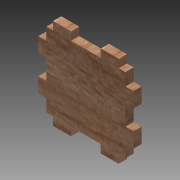
# Autodesk Inventor part: holder_plate_side
Saved by Autodesk Inventor 2015 (Build 190159000, 159)
## iProperties
Created: 2013-12-29
Part Number: holder_plate_side
Material: Wood (Birch)
Document SubType Name: Modeling
Designer: aoki
Density: 1 g/cm^3
Appearance: Birch - Natural Polished
Author: aoki
Autodesk Inventor part; units mm, degrees
ref_plane "YZ Plane" through (0, 0, 0) normal (1, 0, 0) x (0, 1, 0)
ref_plane "XZ Plane" through (0, 0, 0) normal (0, 1, 0) x (-1, 0, 0)
ref_plane "XY Plane" through (0, 0, 0) normal (0, 0, 1) x (1, 0, 0)
sketch "Block1" plane through (0, 0, 0) normal (0, 0, 1) x (1, 0, 0)
  line L0 (-35.5, -12.8333) -> (-26.5, -12.8333)
  line L1 (-30, 3.8333) -> (-35.5, 3.8333)
  line L2 (-35.5, 3.8333) -> (-26.5, 3.8333)
  line L3 (-26.5, 3.8333) -> (-26.5, -12.8333)
  line L4 (-26.5, -12.8333) -> (-35.5, -12.8333)
  line L5 (-35.5, -12.8333) -> (-35.5, 3.8333)
  line L6 (26.5, 3.8333) -> (35.5, 3.8333)
  line L7 (35.5, 3.8333) -> (26.5, 3.8333)
  line L8 (26.5, 3.8333) -> (26.5, -12.8333)
  line L9 (35.5, -12.8333) -> (35.5, 3.8333)
  line L10 (26.5, -12.8333) -> (35.5, -12.8333)
  line L11 (35.5, -12.8333) -> (26.5, -12.8333)
  point P0 (0, -4.5)
  dimension "d37" = 5.5
  measures "d37" distance of L1.start L1.end
sketch "Block2" plane through (0, 0, 0) normal (0, 0, 1) x (1, 0, 0)
  line L0 (-30, -5) -> (-35.5, -5)
  line L1 (-26.5, 5) -> (-35.5, 5)
  line L2 (-35.5, -5) -> (-26.5, -5)
  line L3 (-26.5, -5) -> (-26.5, 5)
  line L4 (-26.5, 5) -> (-35.5, 5)
  line L5 (-35.5, 5) -> (-35.5, -5)
  line L6 (26.5, -5) -> (26.5, 5)
  line L7 (35.5, -5) -> (26.5, -5)
  line L8 (26.5, 5) -> (35.5, 5)
  line L9 (35.5, 5) -> (35.5, -5)
  line L10 (26.5, 5) -> (35.5, 5)
  line L11 (26.5, -5) -> (35.5, -5)
  point P0 (0, 0)
  dimension "d51" = 5.5
  measures "d51" distance of L0.start L0.end
sketch "Block3" plane through (0, 0, 0) normal (0, 0, 1) x (1, 0, 0)
  line L0 (-9.9, 25.1) -> (9.9, 25.1)
  line L1 (9.9, 25.1) -> (9.9, 34.1)
  line L2 (9.9, 34.1) -> (22.1, 34.1)
  line L3 (22.1, 34.1) -> (22.1, 25.1)
  line L4 (22.1, 25.1) -> (26.6, 25.1)
  line L5 (26.6, 25.1) -> (26.6, 16.7667)
  line L6 (26.6, 16.7667) -> (35.6, 16.7667)
  line L7 (35.6, 16.7667) -> (35.6, 6.5667)
  line L8 (35.6, 6.5667) -> (26.6, 6.5667)
  line L9 (26.6, 6.5667) -> (26.6, -6.5667)
  line L10 (26.6, -6.5667) -> (35.6, -6.5667)
  line L11 (35.6, -6.5667) -> (35.6, -16.7667)
  line L12 (35.6, -16.7667) -> (26.6, -16.7667)
  line L13 (26.6, -16.7667) -> (26.6, -25.1)
  line L14 (26.6, -25.1) -> (22.1, -25.1)
  line L15 (22.1, -25.1) -> (22.1, -34.1)
  line L16 (22.1, -34.1) -> (9.9, -34.1)
  line L17 (9.9, -34.1) -> (9.9, -25.1)
  line L18 (9.9, -25.1) -> (-9.9, -25.1)
  line L19 (-9.9, -25.1) -> (-9.9, -34.1)
  line L20 (-9.9, -34.1) -> (-22.1, -34.1)
  line L21 (-22.1, -34.1) -> (-22.1, -25.1)
  line L22 (-22.1, -25.1) -> (-26.6, -25.1)
  line L23 (-26.6, -25.1) -> (-26.6, -16.7667)
  line L24 (-26.6, -16.7667) -> (-35.6, -16.7667)
  line L25 (-35.6, -16.7667) -> (-35.6, -6.5667)
  line L26 (-35.6, -6.5667) -> (-26.6, -6.5667)
  line L27 (-26.6, -6.5667) -> (-26.6, 6.5667)
  line L28 (-26.6, 6.5667) -> (-35.6, 6.5667)
  line L29 (-35.6, 6.5667) -> (-35.6, 16.7667)
  line L30 (-35.6, 16.7667) -> (-26.6, 16.7667)
  line L31 (-26.6, 16.7667) -> (-26.6, 25.1)
  line L32 (-26.6, 25.1) -> (-22.1, 25.1)
  line L33 (-22.1, 25.1) -> (-22.1, 34.1)
  line L34 (-22.1, 34.1) -> (-9.9, 34.1)
  line L35 (-9.9, 34.1) -> (-9.9, 25.1)
  line L36 (-26.5, -6.6667) -> (-35.5, -6.6667)
  line L37 (-35.5, -6.6667) -> (-35.5, -16.6667)
  line L38 (-35.5, -16.6667) -> (-26.5, -16.6667)
  line L39 (-26.5, -16.6667) -> (-26.5, -25)
  line L40 (-26.5, -25) -> (-22, -25)
  line L41 (-22, -25) -> (-22, -34)
  line L42 (-22, -34) -> (-10, -34)
  line L43 (-10, -34) -> (-10, -25)
  line L44 (-10, -25) -> (10, -25)
  line L45 (10, -34) -> (10, -25)
  line L46 (22, -34) -> (10, -34)
  line L47 (22, -25) -> (22, -34)
  line L48 (22, -25) -> (26.5, -25)
  line L49 (26.5, -25) -> (26.5, -16.6667)
  line L50 (26.5, -16.6667) -> (35.5, -16.6667)
  line L51 (35.5, -16.6667) -> (35.5, -6.6667)
  line L52 (35.5, -6.6667) -> (26.5, -6.6667)
  line L53 (26.5, -6.6667) -> (26.5, 6.6667)
  line L54 (26.5, 6.6667) -> (35.5, 6.6667)
  line L55 (35.5, 6.6667) -> (35.5, 16.6667)
  line L56 (35.5, 16.6667) -> (26.5, 16.6667)
  line L57 (26.5, 16.6667) -> (26.5, 25)
  line L58 (26.5, 25) -> (22, 25)
  line L59 (22, 25) -> (22, 34)
  line L60 (22, 34) -> (10, 34)
  line L61 (10, 34) -> (10, 25)
  line L62 (10, 25) -> (-10, 25)
  line L63 (-10, 25) -> (-10, 34)
  line L64 (-10, 34) -> (-22, 34)
  line L65 (-22, 34) -> (-22, 25)
  line L66 (-22, 25) -> (-26.5, 25)
  line L67 (-26.5, 25) -> (-26.5, 16.6667)
  line L68 (-26.5, 16.6667) -> (-35.5, 16.6667)
  line L69 (-35.5, 16.6667) -> (-35.5, 6.6667)
  line L70 (-35.5, 6.6667) -> (-26.5, 6.6667)
  line L71 (-26.5, 6.6667) -> (-26.5, -6.6667)
  line L72 (-9.9, 25.1) -> (9.9, 25.1)
  line L73 (9.9, 25.1) -> (9.9, 34.1)
  line L74 (9.9, 34.1) -> (22.1, 34.1)
  line L75 (22.1, 34.1) -> (22.1, 25.1)
  line L76 (22.1, 25.1) -> (26.6, 25.1)
  line L77 (26.6, 25.1) -> (26.6, 16.7667)
  line L78 (26.6, 16.7667) -> (35.6, 16.7667)
  line L79 (35.6, 16.7667) -> (35.6, 6.5667)
  line L80 (35.6, 6.5667) -> (26.6, 6.5667)
  line L81 (26.6, 6.5667) -> (26.6, -6.5667)
  line L82 (26.6, -6.5667) -> (35.6, -6.5667)
  line L83 (35.6, -6.5667) -> (35.6, -16.7667)
  line L84 (35.6, -16.7667) -> (26.6, -16.7667)
  line L85 (26.6, -16.7667) -> (26.6, -25.1)
  line L86 (26.6, -25.1) -> (22.1, -25.1)
  line L87 (22.1, -25.1) -> (22.1, -34.1)
  line L88 (22.1, -34.1) -> (9.9, -34.1)
  line L89 (9.9, -34.1) -> (9.9, -25.1)
  line L90 (9.9, -25.1) -> (-9.9, -25.1)
  line L91 (-9.9, -25.1) -> (-9.9, -34.1)
  line L92 (-9.9, -34.1) -> (-22.1, -34.1)
  line L93 (-22.1, -34.1) -> (-22.1, -25.1)
  line L94 (-22.1, -25.1) -> (-26.6, -25.1)
  line L95 (-26.6, -25.1) -> (-26.6, -16.7667)
  line L96 (-26.6, -16.7667) -> (-35.6, -16.7667)
  line L97 (-35.6, -16.7667) -> (-35.6, -6.5667)
  line L98 (-35.6, -6.5667) -> (-26.6, -6.5667)
  line L99 (-26.6, -6.5667) -> (-26.6, 6.5667)
  line L100 (-26.6, 6.5667) -> (-35.6, 6.5667)
  line L101 (-35.6, 6.5667) -> (-35.6, 16.7667)
  line L102 (-35.6, 16.7667) -> (-26.6, 16.7667)
  line L103 (-26.6, 16.7667) -> (-26.6, 25.1)
  line L104 (-26.6, 25.1) -> (-22.1, 25.1)
  line L105 (-22.1, 25.1) -> (-22.1, 34.1)
  line L106 (-22.1, 34.1) -> (-9.9, 34.1)
  line L107 (-9.9, 34.1) -> (-9.9, 25.1)
  line L108 (-26.5, -6.6667) -> (-35.5, -6.6667)
  line L109 (-35.5, -6.6667) -> (-35.5, -16.6667)
  line L110 (-35.5, -16.6667) -> (-26.5, -16.6667)
  line L111 (-26.5, -16.6667) -> (-26.5, -25)
  line L112 (-26.5, -25) -> (-22, -25)
  line L113 (-22, -25) -> (-22, -34)
  line L114 (-22, -34) -> (-10, -34)
  line L115 (-10, -34) -> (-10, -25)
  line L116 (-10, -25) -> (10, -25)
  line L117 (10, -34) -> (10, -25)
  line L118 (22, -34) -> (10, -34)
  line L119 (22, -25) -> (22, -34)
  line L120 (22, -25) -> (26.5, -25)
  line L121 (26.5, -25) -> (26.5, -16.6667)
  line L122 (26.5, -16.6667) -> (35.5, -16.6667)
  line L123 (35.5, -16.6667) -> (35.5, -6.6667)
  line L124 (35.5, -6.6667) -> (26.5, -6.6667)
  line L125 (26.5, -6.6667) -> (26.5, 6.6667)
  line L126 (26.5, 6.6667) -> (35.5, 6.6667)
  line L127 (35.5, 6.6667) -> (35.5, 16.6667)
  line L128 (35.5, 16.6667) -> (26.5, 16.6667)
  line L129 (26.5, 16.6667) -> (26.5, 25)
  line L130 (26.5, 25) -> (22, 25)
  line L131 (22, 25) -> (22, 34)
  line L132 (22, 34) -> (10, 34)
  line L133 (10, 34) -> (10, 25)
  line L134 (10, 25) -> (-10, 25)
  line L135 (-10, 25) -> (-10, 34)
  line L136 (-10, 34) -> (-22, 34)
  line L137 (-22, 34) -> (-22, 25)
  line L138 (-22, 25) -> (-26.5, 25)
  line L139 (-26.5, 25) -> (-26.5, 16.6667)
  line L140 (-26.5, 16.6667) -> (-35.5, 16.6667)
  line L141 (-35.5, 16.6667) -> (-35.5, 6.6667)
  line L142 (-35.5, 6.6667) -> (-26.5, 6.6667)
  line L143 (-26.5, 6.6667) -> (-26.5, -6.6667)
  line L144 (-9.9, 25.1) -> (9.9, 25.1)
  line L145 (9.9, 25.1) -> (9.9, 34.1)
  line L146 (9.9, 34.1) -> (22.1, 34.1)
  line L147 (22.1, 34.1) -> (22.1, 25.1)
  line L148 (22.1, 25.1) -> (26.6, 25.1)
  line L149 (26.6, 25.1) -> (26.6, 16.7667)
  line L150 (26.6, 16.7667) -> (35.6, 16.7667)
  line L151 (35.6, 16.7667) -> (35.6, 6.5667)
  line L152 (35.6, 6.5667) -> (26.6, 6.5667)
  line L153 (26.6, 6.5667) -> (26.6, -6.5667)
  line L154 (26.6, -6.5667) -> (35.6, -6.5667)
  line L155 (35.6, -6.5667) -> (35.6, -16.7667)
  line L156 (35.6, -16.7667) -> (26.6, -16.7667)
  line L157 (26.6, -16.7667) -> (26.6, -25.1)
  line L158 (26.6, -25.1) -> (22.1, -25.1)
  line L159 (22.1, -25.1) -> (22.1, -34.1)
  line L160 (22.1, -34.1) -> (9.9, -34.1)
  line L161 (9.9, -34.1) -> (9.9, -25.1)
  line L162 (9.9, -25.1) -> (-9.9, -25.1)
  line L163 (-9.9, -25.1) -> (-9.9, -34.1)
  line L164 (-9.9, -34.1) -> (-22.1, -34.1)
  line L165 (-22.1, -34.1) -> (-22.1, -25.1)
  line L166 (-22.1, -25.1) -> (-26.6, -25.1)
  line L167 (-26.6, -25.1) -> (-26.6, -16.7667)
  line L168 (-26.6, -16.7667) -> (-35.6, -16.7667)
  line L169 (-35.6, -16.7667) -> (-35.6, -6.5667)
  line L170 (-35.6, -6.5667) -> (-26.6, -6.5667)
  line L171 (-26.6, -6.5667) -> (-26.6, 6.5667)
  line L172 (-26.6, 6.5667) -> (-35.6, 6.5667)
  line L173 (-35.6, 6.5667) -> (-35.6, 16.7667)
  line L174 (-35.6, 16.7667) -> (-26.6, 16.7667)
  line L175 (-26.6, 16.7667) -> (-26.6, 25.1)
  line L176 (-26.6, 25.1) -> (-22.1, 25.1)
  line L177 (-22.1, 25.1) -> (-22.1, 34.1)
  line L178 (-22.1, 34.1) -> (-9.9, 34.1)
  line L179 (-9.9, 34.1) -> (-9.9, 25.1)
  line L180 (-26.5, -6.6667) -> (-35.5, -6.6667)
  line L181 (-35.5, -6.6667) -> (-35.5, -16.6667)
  line L182 (-35.5, -16.6667) -> (-26.5, -16.6667)
  line L183 (-26.5, -16.6667) -> (-26.5, -25)
  line L184 (-26.5, -25) -> (-22, -25)
  line L185 (-22, -25) -> (-22, -34)
  line L186 (-22, -34) -> (-10, -34)
  line L187 (-10, -34) -> (-10, -25)
  line L188 (-10, -25) -> (10, -25)
  line L189 (10, -34) -> (10, -25)
  line L190 (22, -34) -> (10, -34)
  line L191 (22, -25) -> (22, -34)
  line L192 (22, -25) -> (26.5, -25)
  line L193 (26.5, -25) -> (26.5, -16.6667)
  line L194 (26.5, -16.6667) -> (35.5, -16.6667)
  line L195 (35.5, -16.6667) -> (35.5, -6.6667)
  line L196 (35.5, -6.6667) -> (26.5, -6.6667)
  line L197 (26.5, -6.6667) -> (26.5, 6.6667)
  line L198 (26.5, 6.6667) -> (35.5, 6.6667)
  line L199 (35.5, 6.6667) -> (35.5, 16.6667)
  line L200 (35.5, 16.6667) -> (26.5, 16.6667)
  line L201 (26.5, 16.6667) -> (26.5, 25)
  line L202 (26.5, 25) -> (22, 25)
  line L203 (22, 25) -> (22, 34)
  line L204 (22, 34) -> (10, 34)
  line L205 (10, 34) -> (10, 25)
  line L206 (10, 25) -> (-10, 25)
  line L207 (-10, 25) -> (-10, 34)
  line L208 (-10, 34) -> (-22, 34)
  line L209 (-22, 34) -> (-22, 25)
  line L210 (-22, 25) -> (-26.5, 25)
  line L211 (-26.5, 25) -> (-26.5, 16.6667)
  line L212 (-26.5, 16.6667) -> (-35.5, 16.6667)
  line L213 (-35.5, 16.6667) -> (-35.5, 6.6667)
  line L214 (-35.5, 6.6667) -> (-26.5, 6.6667)
  line L215 (-26.5, 6.6667) -> (-26.5, -6.6667)
  line L216 (-9.9, 25.1) -> (9.9, 25.1)
  line L217 (9.9, 25.1) -> (9.9, 34.1)
  line L218 (9.9, 34.1) -> (22.1, 34.1)
  line L219 (22.1, 34.1) -> (22.1, 25.1)
  line L220 (22.1, 25.1) -> (26.6, 25.1)
  line L221 (26.6, 25.1) -> (26.6, 16.7667)
  line L222 (26.6, 16.7667) -> (35.6, 16.7667)
  line L223 (35.6, 16.7667) -> (35.6, 6.5667)
  line L224 (35.6, 6.5667) -> (26.6, 6.5667)
  line L225 (26.6, 6.5667) -> (26.6, -6.5667)
  line L226 (26.6, -6.5667) -> (35.6, -6.5667)
  line L227 (35.6, -6.5667) -> (35.6, -16.7667)
  line L228 (35.6, -16.7667) -> (26.6, -16.7667)
  line L229 (26.6, -16.7667) -> (26.6, -25.1)
  line L230 (26.6, -25.1) -> (22.1, -25.1)
  line L231 (22.1, -25.1) -> (22.1, -34.1)
  line L232 (22.1, -34.1) -> (9.9, -34.1)
  line L233 (9.9, -34.1) -> (9.9, -25.1)
  line L234 (9.9, -25.1) -> (-9.9, -25.1)
  line L235 (-9.9, -25.1) -> (-9.9, -34.1)
  line L236 (-9.9, -34.1) -> (-22.1, -34.1)
  line L237 (-22.1, -34.1) -> (-22.1, -25.1)
  line L238 (-22.1, -25.1) -> (-26.6, -25.1)
  line L239 (-26.6, -25.1) -> (-26.6, -16.7667)
  line L240 (-26.6, -16.7667) -> (-35.6, -16.7667)
  line L241 (-35.6, -16.7667) -> (-35.6, -6.5667)
  line L242 (-35.6, -6.5667) -> (-26.6, -6.5667)
  line L243 (-26.6, -6.5667) -> (-26.6, 6.5667)
  line L244 (-26.6, 6.5667) -> (-35.6, 6.5667)
  line L245 (-35.6, 6.5667) -> (-35.6, 16.7667)
  line L246 (-35.6, 16.7667) -> (-26.6, 16.7667)
  line L247 (-26.6, 16.7667) -> (-26.6, 25.1)
  line L248 (-26.6, 25.1) -> (-22.1, 25.1)
  line L249 (-22.1, 25.1) -> (-22.1, 34.1)
  line L250 (-22.1, 34.1) -> (-9.9, 34.1)
  line L251 (-9.9, 34.1) -> (-9.9, 25.1)
  line L252 (-26.5, -6.6667) -> (-35.5, -6.6667)
  line L253 (-35.5, -6.6667) -> (-35.5, -16.6667)
  line L254 (-35.5, -16.6667) -> (-26.5, -16.6667)
  line L255 (-26.5, -16.6667) -> (-26.5, -25)
  line L256 (-26.5, -25) -> (-22, -25)
  line L257 (-22, -25) -> (-22, -34)
  line L258 (-22, -34) -> (-10, -34)
  line L259 (-10, -34) -> (-10, -25)
  line L260 (-10, -25) -> (10, -25)
  line L261 (10, -34) -> (10, -25)
  line L262 (22, -34) -> (10, -34)
  line L263 (22, -25) -> (22, -34)
  line L264 (22, -25) -> (26.5, -25)
  line L265 (26.5, -25) -> (26.5, -16.6667)
  line L266 (26.5, -16.6667) -> (35.5, -16.6667)
  line L267 (35.5, -16.6667) -> (35.5, -6.6667)
  line L268 (35.5, -6.6667) -> (26.5, -6.6667)
  line L269 (26.5, -6.6667) -> (26.5, 6.6667)
  line L270 (26.5, 6.6667) -> (35.5, 6.6667)
  line L271 (35.5, 6.6667) -> (35.5, 16.6667)
  line L272 (35.5, 16.6667) -> (26.5, 16.6667)
  line L273 (26.5, 16.6667) -> (26.5, 25)
  line L274 (26.5, 25) -> (22, 25)
  line L275 (22, 25) -> (22, 34)
  line L276 (22, 34) -> (10, 34)
  line L277 (10, 34) -> (10, 25)
  line L278 (10, 25) -> (-10, 25)
  line L279 (-10, 25) -> (-10, 34)
  line L280 (-10, 34) -> (-22, 34)
  line L281 (-22, 34) -> (-22, 25)
  line L282 (-22, 25) -> (-26.5, 25)
  line L283 (-26.5, 25) -> (-26.5, 16.6667)
  line L284 (-26.5, 16.6667) -> (-35.5, 16.6667)
  line L285 (-35.5, 16.6667) -> (-35.5, 6.6667)
  line L286 (-35.5, 6.6667) -> (-26.5, 6.6667)
  line L287 (-26.5, 6.6667) -> (-26.5, -6.6667)
  line L288 (-9.9, 25.1) -> (9.9, 25.1)
  line L289 (9.9, 25.1) -> (9.9, 34.1)
  line L290 (9.9, 34.1) -> (22.1, 34.1)
  line L291 (22.1, 34.1) -> (22.1, 25.1)
  line L292 (22.1, 25.1) -> (26.6, 25.1)
  line L293 (26.6, 25.1) -> (26.6, 16.7667)
  line L294 (26.6, 16.7667) -> (35.6, 16.7667)
  line L295 (35.6, 16.7667) -> (35.6, 6.5667)
  line L296 (35.6, 6.5667) -> (26.6, 6.5667)
  line L297 (26.6, 6.5667) -> (26.6, -6.5667)
  line L298 (26.6, -6.5667) -> (35.6, -6.5667)
  line L299 (35.6, -6.5667) -> (35.6, -16.7667)
  line L300 (35.6, -16.7667) -> (26.6, -16.7667)
  line L301 (26.6, -16.7667) -> (26.6, -25.1)
  line L302 (26.6, -25.1) -> (22.1, -25.1)
  line L303 (22.1, -25.1) -> (22.1, -34.1)
  line L304 (22.1, -34.1) -> (9.9, -34.1)
  line L305 (9.9, -34.1) -> (9.9, -25.1)
  line L306 (9.9, -25.1) -> (-9.9, -25.1)
  line L307 (-9.9, -25.1) -> (-9.9, -34.1)
  line L308 (-9.9, -34.1) -> (-22.1, -34.1)
  line L309 (-22.1, -34.1) -> (-22.1, -25.1)
  line L310 (-22.1, -25.1) -> (-26.6, -25.1)
  line L311 (-26.6, -25.1) -> (-26.6, -16.7667)
  line L312 (-26.6, -16.7667) -> (-35.6, -16.7667)
  line L313 (-35.6, -16.7667) -> (-35.6, -6.5667)
  line L314 (-35.6, -6.5667) -> (-26.6, -6.5667)
  line L315 (-26.6, -6.5667) -> (-26.6, 6.5667)
  line L316 (-26.6, 6.5667) -> (-35.6, 6.5667)
  line L317 (-35.6, 6.5667) -> (-35.6, 16.7667)
  line L318 (-35.6, 16.7667) -> (-26.6, 16.7667)
  line L319 (-26.6, 16.7667) -> (-26.6, 25.1)
  line L320 (-26.6, 25.1) -> (-22.1, 25.1)
  line L321 (-22.1, 25.1) -> (-22.1, 34.1)
  line L322 (-22.1, 34.1) -> (-9.9, 34.1)
  line L323 (-9.9, 34.1) -> (-9.9, 25.1)
  line L324 (-26.5, -6.6667) -> (-35.5, -6.6667)
  line L325 (-35.5, -6.6667) -> (-35.5, -16.6667)
  line L326 (-35.5, -16.6667) -> (-26.5, -16.6667)
  line L327 (-26.5, -16.6667) -> (-26.5, -25)
  line L328 (-26.5, -25) -> (-22, -25)
  line L329 (-22, -25) -> (-22, -34)
  line L330 (-22, -34) -> (-10, -34)
  line L331 (-10, -34) -> (-10, -25)
  line L332 (-10, -25) -> (10, -25)
  line L333 (10, -34) -> (10, -25)
  line L334 (22, -34) -> (10, -34)
  line L335 (22, -25) -> (22, -34)
  line L336 (22, -25) -> (26.5, -25)
  line L337 (26.5, -25) -> (26.5, -16.6667)
  line L338 (26.5, -16.6667) -> (35.5, -16.6667)
  line L339 (35.5, -16.6667) -> (35.5, -6.6667)
  line L340 (35.5, -6.6667) -> (26.5, -6.6667)
  line L341 (26.5, -6.6667) -> (26.5, 6.6667)
  line L342 (26.5, 6.6667) -> (35.5, 6.6667)
  line L343 (35.5, 6.6667) -> (35.5, 16.6667)
  line L344 (35.5, 16.6667) -> (26.5, 16.6667)
  line L345 (26.5, 16.6667) -> (26.5, 25)
  line L346 (26.5, 25) -> (22, 25)
  line L347 (22, 25) -> (22, 34)
  line L348 (22, 34) -> (10, 34)
  line L349 (10, 34) -> (10, 25)
  line L350 (10, 25) -> (-10, 25)
  line L351 (-10, 25) -> (-10, 34)
  line L352 (-10, 34) -> (-22, 34)
  line L353 (-22, 34) -> (-22, 25)
  line L354 (-22, 25) -> (-26.5, 25)
  line L355 (-26.5, 25) -> (-26.5, 16.6667)
  line L356 (-26.5, 16.6667) -> (-35.5, 16.6667)
  line L357 (-35.5, 16.6667) -> (-35.5, 6.6667)
  line L358 (-35.5, 6.6667) -> (-26.5, 6.6667)
  line L359 (-26.5, 6.6667) -> (-26.5, -6.6667)
  line L360 (-9.9, 25.1) -> (9.9, 25.1)
  line L361 (9.9, 25.1) -> (9.9, 34.1)
  line L362 (9.9, 34.1) -> (22.1, 34.1)
  line L363 (22.1, 34.1) -> (22.1, 25.1)
  line L364 (22.1, 25.1) -> (26.6, 25.1)
  line L365 (26.6, 25.1) -> (26.6, 16.7667)
  line L366 (26.6, 16.7667) -> (35.6, 16.7667)
  line L367 (35.6, 16.7667) -> (35.6, 6.5667)
  line L368 (35.6, 6.5667) -> (26.6, 6.5667)
  line L369 (26.6, 6.5667) -> (26.6, -6.5667)
  line L370 (26.6, -6.5667) -> (35.6, -6.5667)
  line L371 (35.6, -6.5667) -> (35.6, -16.7667)
  line L372 (35.6, -16.7667) -> (26.6, -16.7667)
  line L373 (26.6, -16.7667) -> (26.6, -25.1)
  line L374 (26.6, -25.1) -> (22.1, -25.1)
  line L375 (22.1, -25.1) -> (22.1, -34.1)
  line L376 (22.1, -34.1) -> (9.9, -34.1)
  line L377 (9.9, -34.1) -> (9.9, -25.1)
  line L378 (9.9, -25.1) -> (-9.9, -25.1)
  line L379 (-9.9, -25.1) -> (-9.9, -34.1)
  line L380 (-9.9, -34.1) -> (-22.1, -34.1)
  line L381 (-22.1, -34.1) -> (-22.1, -25.1)
  line L382 (-22.1, -25.1) -> (-26.6, -25.1)
  line L383 (-26.6, -25.1) -> (-26.6, -16.7667)
  line L384 (-26.6, -16.7667) -> (-35.6, -16.7667)
  line L385 (-35.6, -16.7667) -> (-35.6, -6.5667)
  line L386 (-35.6, -6.5667) -> (-26.6, -6.5667)
  line L387 (-26.6, -6.5667) -> (-26.6, 6.5667)
  line L388 (-26.6, 6.5667) -> (-35.6, 6.5667)
  line L389 (-35.6, 6.5667) -> (-35.6, 16.7667)
  line L390 (-35.6, 16.7667) -> (-26.6, 16.7667)
  line L391 (-26.6, 16.7667) -> (-26.6, 25.1)
  line L392 (-26.6, 25.1) -> (-22.1, 25.1)
  line L393 (-22.1, 25.1) -> (-22.1, 34.1)
  line L394 (-22.1, 34.1) -> (-9.9, 34.1)
  line L395 (-9.9, 34.1) -> (-9.9, 25.1)
  line L396 (-26.5, -6.6667) -> (-35.5, -6.6667)
  line L397 (-35.5, -6.6667) -> (-35.5, -16.6667)
  line L398 (-35.5, -16.6667) -> (-26.5, -16.6667)
  line L399 (-26.5, -16.6667) -> (-26.5, -25)
  line L400 (-26.5, -25) -> (-22, -25)
  line L401 (-22, -25) -> (-22, -34)
  line L402 (-22, -34) -> (-10, -34)
  line L403 (-10, -34) -> (-10, -25)
  line L404 (-10, -25) -> (10, -25)
  line L405 (10, -34) -> (10, -25)
  line L406 (22, -34) -> (10, -34)
  line L407 (22, -25) -> (22, -34)
  line L408 (22, -25) -> (26.5, -25)
  line L409 (26.5, -25) -> (26.5, -16.6667)
  line L410 (26.5, -16.6667) -> (35.5, -16.6667)
  line L411 (35.5, -16.6667) -> (35.5, -6.6667)
  line L412 (35.5, -6.6667) -> (26.5, -6.6667)
  line L413 (26.5, -6.6667) -> (26.5, 6.6667)
  line L414 (26.5, 6.6667) -> (35.5, 6.6667)
  line L415 (35.5, 6.6667) -> (35.5, 16.6667)
  line L416 (35.5, 16.6667) -> (26.5, 16.6667)
  line L417 (26.5, 16.6667) -> (26.5, 25)
  line L418 (26.5, 25) -> (22, 25)
  line L419 (22, 25) -> (22, 34)
  line L420 (22, 34) -> (10, 34)
  line L421 (10, 34) -> (10, 25)
  line L422 (10, 25) -> (-10, 25)
  line L423 (-10, 25) -> (-10, 34)
  line L424 (-10, 34) -> (-22, 34)
  line L425 (-22, 34) -> (-22, 25)
  line L426 (-22, 25) -> (-26.5, 25)
  line L427 (-26.5, 25) -> (-26.5, 16.6667)
  line L428 (-26.5, 16.6667) -> (-35.5, 16.6667)
  line L429 (-35.5, 16.6667) -> (-35.5, 6.6667)
  line L430 (-35.5, 6.6667) -> (-26.5, 6.6667)
  line L431 (-26.5, 6.6667) -> (-26.5, -6.6667)
  line L432 (-9.9, 25.1) -> (9.9, 25.1)
  line L433 (9.9, 25.1) -> (9.9, 34.1)
  line L434 (9.9, 34.1) -> (22.1, 34.1)
  line L435 (22.1, 34.1) -> (22.1, 25.1)
  line L436 (22.1, 25.1) -> (26.6, 25.1)
  line L437 (26.6, 25.1) -> (26.6, 16.7667)
  line L438 (26.6, 16.7667) -> (35.6, 16.7667)
  line L439 (35.6, 16.7667) -> (35.6, 6.5667)
  line L440 (35.6, 6.5667) -> (26.6, 6.5667)
  line L441 (26.6, 6.5667) -> (26.6, -6.5667)
  line L442 (26.6, -6.5667) -> (35.6, -6.5667)
  line L443 (35.6, -6.5667) -> (35.6, -16.7667)
  line L444 (35.6, -16.7667) -> (26.6, -16.7667)
  line L445 (26.6, -16.7667) -> (26.6, -25.1)
  line L446 (26.6, -25.1) -> (22.1, -25.1)
  line L447 (22.1, -25.1) -> (22.1, -34.1)
  line L448 (22.1, -34.1) -> (9.9, -34.1)
  line L449 (9.9, -34.1) -> (9.9, -25.1)
  line L450 (9.9, -25.1) -> (-9.9, -25.1)
  line L451 (-9.9, -25.1) -> (-9.9, -34.1)
  line L452 (-9.9, -34.1) -> (-22.1, -34.1)
  line L453 (-22.1, -34.1) -> (-22.1, -25.1)
  line L454 (-22.1, -25.1) -> (-26.6, -25.1)
  line L455 (-26.6, -25.1) -> (-26.6, -16.7667)
  line L456 (-26.6, -16.7667) -> (-35.6, -16.7667)
  line L457 (-35.6, -16.7667) -> (-35.6, -6.5667)
  line L458 (-35.6, -6.5667) -> (-26.6, -6.5667)
  line L459 (-26.6, -6.5667) -> (-26.6, 6.5667)
  line L460 (-26.6, 6.5667) -> (-35.6, 6.5667)
  line L461 (-35.6, 6.5667) -> (-35.6, 16.7667)
  line L462 (-35.6, 16.7667) -> (-26.6, 16.7667)
  line L463 (-26.6, 16.7667) -> (-26.6, 25.1)
  line L464 (-26.6, 25.1) -> (-22.1, 25.1)
  line L465 (-22.1, 25.1) -> (-22.1, 34.1)
  line L466 (-22.1, 34.1) -> (-9.9, 34.1)
  line L467 (-9.9, 34.1) -> (-9.9, 25.1)
  line L468 (-26.5, -6.6667) -> (-35.5, -6.6667)
  line L469 (-35.5, -6.6667) -> (-35.5, -16.6667)
  line L470 (-35.5, -16.6667) -> (-26.5, -16.6667)
  line L471 (-26.5, -16.6667) -> (-26.5, -25)
  line L472 (-26.5, -25) -> (-22, -25)
  line L473 (-22, -25) -> (-22, -34)
  line L474 (-22, -34) -> (-10, -34)
  line L475 (-10, -34) -> (-10, -25)
  line L476 (-10, -25) -> (10, -25)
  line L477 (10, -34) -> (10, -25)
  line L478 (22, -34) -> (10, -34)
  line L479 (22, -25) -> (22, -34)
  line L480 (22, -25) -> (26.5, -25)
  line L481 (26.5, -25) -> (26.5, -16.6667)
  line L482 (26.5, -16.6667) -> (35.5, -16.6667)
  line L483 (35.5, -16.6667) -> (35.5, -6.6667)
  line L484 (35.5, -6.6667) -> (26.5, -6.6667)
  line L485 (26.5, -6.6667) -> (26.5, 6.6667)
  line L486 (26.5, 6.6667) -> (35.5, 6.6667)
  line L487 (35.5, 6.6667) -> (35.5, 16.6667)
  line L488 (35.5, 16.6667) -> (26.5, 16.6667)
  line L489 (26.5, 16.6667) -> (26.5, 25)
  line L490 (26.5, 25) -> (22, 25)
  line L491 (22, 25) -> (22, 34)
  line L492 (22, 34) -> (10, 34)
  line L493 (10, 34) -> (10, 25)
  line L494 (10, 25) -> (-10, 25)
  line L495 (-10, 25) -> (-10, 34)
  line L496 (-10, 34) -> (-22, 34)
  line L497 (-22, 34) -> (-22, 25)
  line L498 (-22, 25) -> (-26.5, 25)
  line L499 (-26.5, 25) -> (-26.5, 16.6667)
  line L500 (-26.5, 16.6667) -> (-35.5, 16.6667)
  line L501 (-35.5, 16.6667) -> (-35.5, 6.6667)
  line L502 (-35.5, 6.6667) -> (-26.5, 6.6667)
  line L503 (-26.5, 6.6667) -> (-26.5, -6.6667)
  line L504 (-9.9, 25.1) -> (9.9, 25.1)
  line L505 (9.9, 25.1) -> (9.9, 34.1)
  line L506 (9.9, 34.1) -> (22.1, 34.1)
  line L507 (22.1, 34.1) -> (22.1, 25.1)
  line L508 (22.1, 25.1) -> (26.6, 25.1)
  line L509 (26.6, 25.1) -> (26.6, 16.7667)
  line L510 (26.6, 16.7667) -> (35.6, 16.7667)
  line L511 (35.6, 16.7667) -> (35.6, 6.5667)
  line L512 (35.6, 6.5667) -> (26.6, 6.5667)
  line L513 (26.6, 6.5667) -> (26.6, -6.5667)
  line L514 (26.6, -6.5667) -> (35.6, -6.5667)
  line L515 (35.6, -6.5667) -> (35.6, -16.7667)
  line L516 (35.6, -16.7667) -> (26.6, -16.7667)
  line L517 (26.6, -16.7667) -> (26.6, -25.1)
  line L518 (26.6, -25.1) -> (22.1, -25.1)
  line L519 (22.1, -25.1) -> (22.1, -34.1)
  line L520 (22.1, -34.1) -> (9.9, -34.1)
  line L521 (9.9, -34.1) -> (9.9, -25.1)
  line L522 (9.9, -25.1) -> (-9.9, -25.1)
  line L523 (-9.9, -25.1) -> (-9.9, -34.1)
  line L524 (-9.9, -34.1) -> (-22.1, -34.1)
  line L525 (-22.1, -34.1) -> (-22.1, -25.1)
  line L526 (-22.1, -25.1) -> (-26.6, -25.1)
  line L527 (-26.6, -25.1) -> (-26.6, -16.7667)
  line L528 (-26.6, -16.7667) -> (-35.6, -16.7667)
  line L529 (-35.6, -16.7667) -> (-35.6, -6.5667)
  line L530 (-35.6, -6.5667) -> (-26.6, -6.5667)
  line L531 (-26.6, -6.5667) -> (-26.6, 6.5667)
  line L532 (-26.6, 6.5667) -> (-35.6, 6.5667)
  line L533 (-35.6, 6.5667) -> (-35.6, 16.7667)
  line L534 (-35.6, 16.7667) -> (-26.6, 16.7667)
  line L535 (-26.6, 16.7667) -> (-26.6, 25.1)
  line L536 (-26.6, 25.1) -> (-22.1, 25.1)
  line L537 (-22.1, 25.1) -> (-22.1, 34.1)
  line L538 (-22.1, 34.1) -> (-9.9, 34.1)
  line L539 (-9.9, 34.1) -> (-9.9, 25.1)
  point P0 (0, 0)
  point P1 (0, 0)
  point P2 (0, 0)
  point P3 (0, 0)
  point P4 (0, 0)
  point P5 (0, 0)
  point P6 (0, 0)
  point P7 (0, 0)
  dimension "d58" = 0.1
  dimension "d60" = 0.1
  dimension "d61" = 0.1
  dimension "d64" = 0.1
  dimension "d65" = 0.1
  dimension "d66" = 0.1
  dimension "d67" = 0.1
  measures "d58" distance between parallel lines of L72 L62
  measures "d60" distance between parallel lines of L144 L134
  measures "d61" distance between parallel lines of L216 L206
  measures "d64" distance between parallel lines of L288 L278
  measures "d65" distance between parallel lines of L360 L350
  measures "d66" distance between parallel lines of L432 L422
  measures "d67" distance between parallel lines of L504 L494
sketch "Block4" plane through (0, 0, 0) normal (0, 0, 1) x (1, 0, 0)
  line L0 (-8, 27) -> (8, 27)
  line L1 (8, 27) -> (8, 36)
  line L2 (8, 36) -> (24, 36)
  line L3 (24, 36) -> (24, 27)
  line L4 (24, 27) -> (28.5, 27)
  line L5 (28.5, 27) -> (28.5, 18.6667)
  line L6 (28.5, 18.6667) -> (37.5, 18.6667)
  line L7 (37.5, 18.6667) -> (37.5, 4.6667)
  line L8 (37.5, 4.6667) -> (28.5, 4.6667)
  line L9 (28.5, 4.6667) -> (28.5, -4.6667)
  line L10 (28.5, -4.6667) -> (37.5, -4.6667)
  line L11 (37.5, -4.6667) -> (37.5, -18.6667)
  line L12 (37.5, -18.6667) -> (28.5, -18.6667)
  line L13 (28.5, -18.6667) -> (28.5, -27)
  line L14 (28.5, -27) -> (24, -27)
  line L15 (24, -27) -> (24, -36)
  line L16 (24, -36) -> (8, -36)
  line L17 (8, -36) -> (8, -27)
  line L18 (8, -27) -> (-8, -27)
  line L19 (-8, -27) -> (-8, -36)
  line L20 (-8, -36) -> (-24, -36)
  line L21 (-24, -36) -> (-24, -27)
  line L22 (-24, -27) -> (-28.5, -27)
  line L23 (-28.5, -27) -> (-28.5, -18.6667)
  line L24 (-28.5, -18.6667) -> (-37.5, -18.6667)
  line L25 (-37.5, -18.6667) -> (-37.5, -4.6667)
  line L26 (-37.5, -4.6667) -> (-28.5, -4.6667)
  line L27 (-28.5, -4.6667) -> (-28.5, 4.6667)
  line L28 (-28.5, 4.6667) -> (-37.5, 4.6667)
  line L29 (-37.5, 4.6667) -> (-37.5, 18.6667)
  line L30 (-37.5, 18.6667) -> (-28.5, 18.6667)
  line L31 (-28.5, 18.6667) -> (-28.5, 27)
  line L32 (-28.5, 27) -> (-24, 27)
  line L33 (-24, 27) -> (-24, 36)
  line L34 (-24, 36) -> (-8, 36)
  line L35 (-8, 36) -> (-8, 27)
  point P0 (0, 0)
sketch "Block5" plane through (0, 0, 0) normal (0, 0, 1) x (1, 0, 0)
  line L0 (-9.9, 25.1) -> (9.9, 25.1)
  line L1 (9.9, 25.1) -> (9.9, 34.1)
  line L2 (9.9, 34.1) -> (22.1, 34.1)
  line L3 (22.1, 34.1) -> (22.1, 25.1)
  line L4 (22.1, 25.1) -> (26.6, 25.1)
  line L5 (26.6, 25.1) -> (26.6, 16.7667)
  line L6 (26.6, 16.7667) -> (35.6, 16.7667)
  line L7 (35.6, 16.7667) -> (35.6, 6.5667)
  line L8 (35.6, 6.5667) -> (26.6, 6.5667)
  line L9 (26.6, 6.5667) -> (26.6, -6.5667)
  line L10 (26.6, -6.5667) -> (35.6, -6.5667)
  line L11 (35.6, -6.5667) -> (35.6, -16.7667)
  line L12 (35.6, -16.7667) -> (26.6, -16.7667)
  line L13 (26.6, -16.7667) -> (26.6, -25.1)
  line L14 (26.6, -25.1) -> (22.1, -25.1)
  line L15 (22.1, -25.1) -> (22.1, -34.1)
  line L16 (22.1, -34.1) -> (9.9, -34.1)
  line L17 (9.9, -34.1) -> (9.9, -25.1)
  line L18 (9.9, -25.1) -> (-9.9, -25.1)
  line L19 (-9.9, -25.1) -> (-9.9, -34.1)
  line L20 (-9.9, -34.1) -> (-22.1, -34.1)
  line L21 (-22.1, -34.1) -> (-22.1, -25.1)
  line L22 (-22.1, -25.1) -> (-26.6, -25.1)
  line L23 (-26.6, -25.1) -> (-26.6, -16.7667)
  line L24 (-26.6, -16.7667) -> (-35.6, -16.7667)
  line L25 (-35.6, -16.7667) -> (-35.6, -6.5667)
  line L26 (-35.6, -6.5667) -> (-26.6, -6.5667)
  line L27 (-26.6, -6.5667) -> (-26.6, 6.5667)
  line L28 (-26.6, 6.5667) -> (-35.6, 6.5667)
  line L29 (-35.6, 6.5667) -> (-35.6, 16.7667)
  line L30 (-35.6, 16.7667) -> (-26.6, 16.7667)
  line L31 (-26.6, 16.7667) -> (-26.6, 25.1)
  line L32 (-26.6, 25.1) -> (-22.1, 25.1)
  line L33 (-22.1, 25.1) -> (-22.1, 34.1)
  line L34 (-22.1, 34.1) -> (-9.9, 34.1)
  line L35 (-9.9, 34.1) -> (-9.9, 25.1)
  point P0 (0, 0)
sketch "Block6" plane through (0, 0, 0) normal (0, 0, 1) x (1, 0, 0)
  line L0 (9.8, 34.2) -> (22.2, 34.2)
  line L1 (22.2, 34.2) -> (22.2, 25.2)
  line L2 (22.2, 25.2) -> (26.7, 25.2)
  line L3 (26.7, 25.2) -> (26.7, 16.8667)
  line L4 (26.7, 16.8667) -> (35.7, 16.8667)
  line L5 (35.7, 16.8667) -> (35.7, 6.4667)
  line L6 (35.7, 6.4667) -> (26.7, 6.4667)
  line L7 (26.7, 6.4667) -> (26.7, -6.4667)
  line L8 (26.7, -6.4667) -> (35.7, -6.4667)
  line L9 (35.7, -6.4667) -> (35.7, -16.8667)
  line L10 (35.7, -16.8667) -> (26.7, -16.8667)
  line L11 (26.7, -16.8667) -> (26.7, -25.2)
  line L12 (26.7, -25.2) -> (22.2, -25.2)
  line L13 (22.2, -25.2) -> (22.2, -34.2)
  line L14 (22.2, -34.2) -> (9.8, -34.2)
  line L15 (9.8, -34.2) -> (9.8, -25.2)
  line L16 (9.8, -25.2) -> (-9.8, -25.2)
  line L17 (-9.8, -25.2) -> (-9.8, -34.2)
  line L18 (-9.8, -34.2) -> (-22.2, -34.2)
  line L19 (-22.2, -34.2) -> (-22.2, -25.2)
  line L20 (-22.2, -25.2) -> (-26.7, -25.2)
  line L21 (-26.7, -25.2) -> (-26.7, -16.8667)
  line L22 (-26.7, -16.8667) -> (-35.7, -16.8667)
  line L23 (-35.7, -16.8667) -> (-35.7, -6.4667)
  line L24 (-35.7, -6.4667) -> (-26.7, -6.4667)
  line L25 (-26.7, -6.4667) -> (-26.7, 6.4667)
  line L26 (-26.7, 6.4667) -> (-35.7, 6.4667)
  line L27 (-35.7, 6.4667) -> (-35.7, 16.8667)
  line L28 (-35.7, 16.8667) -> (-26.7, 16.8667)
  line L29 (-26.7, 16.8667) -> (-26.7, 25.2)
  line L30 (-26.7, 25.2) -> (-22.2, 25.2)
  line L31 (-22.2, 25.2) -> (-22.2, 34.2)
  line L32 (-22.2, 34.2) -> (-9.8, 34.2)
  line L33 (-9.8, 34.2) -> (-9.8, 25.2)
  line L34 (-9.8, 25.2) -> (9.8, 25.2)
  line L35 (9.8, 25.2) -> (9.8, 34.2)
  point P0 (0, 0)
sketch "Block7" plane through (0, 0, 0) normal (0, 0, 1) x (1, 0, 0)
  line L0 (9.9, 34.1) -> (22.1, 34.1)
  line L1 (22.1, 34.1) -> (22.1, 25.1)
  line L2 (22.1, 25.1) -> (26.6, 25.1)
  line L3 (26.6, 25.1) -> (26.6, 16.7667)
  line L4 (26.6, 16.7667) -> (35.6, 16.7667)
  line L5 (35.6, 16.7667) -> (35.6, 6.5667)
  line L6 (35.6, 6.5667) -> (26.6, 6.5667)
  line L7 (26.6, 6.5667) -> (26.6, -6.5667)
  line L8 (26.6, -6.5667) -> (35.6, -6.5667)
  line L9 (35.6, -6.5667) -> (35.6, -16.7667)
  line L10 (35.6, -16.7667) -> (26.6, -16.7667)
  line L11 (26.6, -16.7667) -> (26.6, -25.1)
  line L12 (26.6, -25.1) -> (22.1, -25.1)
  line L13 (22.1, -25.1) -> (22.1, -34.1)
  line L14 (22.1, -34.1) -> (9.9, -34.1)
  line L15 (9.9, -34.1) -> (9.9, -25.1)
  line L16 (9.9, -25.1) -> (-9.9, -25.1)
  line L17 (-9.9, -25.1) -> (-9.9, -34.1)
  line L18 (-9.9, -34.1) -> (-22.1, -34.1)
  line L19 (-22.1, -34.1) -> (-22.1, -25.1)
  line L20 (-22.1, -25.1) -> (-26.6, -25.1)
  line L21 (-26.6, -25.1) -> (-26.6, -16.7667)
  line L22 (-26.6, -16.7667) -> (-35.6, -16.7667)
  line L23 (-35.6, -16.7667) -> (-35.6, -6.5667)
  line L24 (-35.6, -6.5667) -> (-26.6, -6.5667)
  line L25 (-26.6, -6.5667) -> (-26.6, 6.5667)
  line L26 (-26.6, 6.5667) -> (-35.6, 6.5667)
  line L27 (-35.6, 6.5667) -> (-35.6, 16.7667)
  line L28 (-35.6, 16.7667) -> (-26.6, 16.7667)
  line L29 (-26.6, 16.7667) -> (-26.6, 25.1)
  line L30 (-26.6, 25.1) -> (-22.1, 25.1)
  line L31 (-22.1, 25.1) -> (-22.1, 34.1)
  line L32 (-22.1, 34.1) -> (-9.9, 34.1)
  line L33 (-9.9, 34.1) -> (-9.9, 25.1)
  line L34 (-9.9, 25.1) -> (9.9, 25.1)
  line L35 (9.9, 25.1) -> (9.9, 34.1)
  point P0 (0, 0)
sketch "Block8" plane through (0, 0, 0) normal (0, 0, 1) x (1, 0, 0)
  line L0 (-9.92, 25.08) -> (9.92, 25.08)
  line L1 (9.92, 25.08) -> (9.92, 30.58)
  line L2 (9.92, 30.58) -> (22.08, 30.58)
  line L3 (22.08, 30.58) -> (22.08, 25.08)
  line L4 (22.08, 25.08) -> (26.58, 25.08)
  line L5 (26.58, 25.08) -> (26.58, 16.7467)
  line L6 (26.58, 16.7467) -> (32.08, 16.7467)
  line L7 (32.08, 16.7467) -> (32.08, 6.5867)
  line L8 (32.08, 6.5867) -> (26.58, 6.5867)
  line L9 (26.58, 6.5867) -> (26.58, -6.5867)
  line L10 (26.58, -6.5867) -> (32.08, -6.5867)
  line L11 (32.08, -6.5867) -> (32.08, -16.7467)
  line L12 (32.08, -16.7467) -> (26.58, -16.7467)
  line L13 (26.58, -16.7467) -> (26.58, -25.08)
  line L14 (26.58, -25.08) -> (22.08, -25.08)
  line L15 (22.08, -25.08) -> (22.08, -30.58)
  line L16 (22.08, -30.58) -> (9.92, -30.58)
  line L17 (9.92, -30.58) -> (9.92, -25.08)
  line L18 (9.92, -25.08) -> (-9.92, -25.08)
  line L19 (-9.92, -25.08) -> (-9.92, -30.58)
  line L20 (-9.92, -30.58) -> (-22.08, -30.58)
  line L21 (-22.08, -30.58) -> (-22.08, -25.08)
  line L22 (-22.08, -25.08) -> (-26.58, -25.08)
  line L23 (-26.58, -25.08) -> (-26.58, -16.7467)
  line L24 (-26.58, -16.7467) -> (-32.08, -16.7467)
  line L25 (-32.08, -16.7467) -> (-32.08, -6.5867)
  line L26 (-32.08, -6.5867) -> (-26.58, -6.5867)
  line L27 (-26.58, -6.5867) -> (-26.58, 6.5867)
  line L28 (-26.58, 6.5867) -> (-32.08, 6.5867)
  line L29 (-32.08, 6.5867) -> (-32.08, 16.7467)
  line L30 (-32.08, 16.7467) -> (-26.58, 16.7467)
  line L31 (-26.58, 16.7467) -> (-26.58, 25.08)
  line L32 (-26.58, 25.08) -> (-22.08, 25.08)
  line L33 (-22.08, 25.08) -> (-22.08, 30.58)
  line L34 (-22.08, 30.58) -> (-9.92, 30.58)
  line L35 (-9.92, 30.58) -> (-9.92, 25.08)
  point P0 (0, 0)
sketch "Sketch2" plane through (0, 0, 0) normal (0, 1, 0) x (-1, 0, 0)
  line L0 (32, -25) -> (-32, -25)
  line L1 (-32, -25) -> (-32, 25)
  line L2 (-32, 25) -> (32, 25)
  line L3 (32, 25) -> (32, -25)
  line L4 (32, -25) -> (-32, 25) construction
  line L5 (-32, -25) -> (32, 25) construction
  point P0 (0, 0)
  dimension "d0" = 64
  dimension "d1" = 50
  constraints: 12 end point, 2 midpoint, 2 parallel, 1 horizontal, 1 perpendicular
  measures "d0" distance of L1.end L2.end
  measures "d1" distance of L0.end L1.end
extrude "Extrusion1" add sketch "Sketch2" along normal blind 5.5
sketch "Sketch4" plane through (0, 0, 0) normal (0, -1, 0) x (1, 0, 0)
  line L0 (-32, -25) -> (32, -25) projected
  line L1 (-22, -25) -> (-10, -25)
  line L2 (-10, -25) -> (-10, -30.5)
  line L3 (-10, -30.5) -> (-22, -30.5)
  line L4 (-22, -30.5) -> (-22, -25)
  line L5 (0, -47.9488) -> (0, 48.9927) projected
  line L6 (-1026.854, 0) -> (1026.854, 0) projected
  line L7 (22, -25) -> (10, -25)
  line L8 (10, -25) -> (10, -30.5)
  line L9 (10, -30.5) -> (22, -30.5)
  line L10 (22, -30.5) -> (22, -25)
  line L11 (-22, 25) -> (-10, 25)
  line L12 (-10, 25) -> (-10, 30.5)
  line L13 (-10, 30.5) -> (-22, 30.5)
  line L14 (-22, 30.5) -> (-22, 25)
  line L15 (10, 25) -> (10, 30.5)
  line L16 (10, 30.5) -> (22, 30.5)
  line L17 (22, 30.5) -> (22, 25)
  line L18 (22, 25) -> (10, 25)
  point P0 (0, 0)
  dimension "d9" = 5.5
  dimension "d10" = 20
  dimension "d11" = 12
  constraints: 32 end point, 12 symmetric about line, 2 parallel, 1 horizontal, 1 perpendicular, 1 point on line
  measures "d9" distance of L3.end L1.start
  measures "d10" distance between parallel lines of L8 L2
  measures "d11" distance of L2.end L3.end
extrude "Extrusion3" add sketch "Sketch4" against normal blind 5.5
sketch "Sketch7" plane through (0, 5.5, 0) normal (0, 1, 0) x (1, 0, 0)
  line L0 (0, 47.9488) -> (0, -48.9927) projected
  line L1 (-32, -25) -> (-26.5, -25)
  line L2 (-26.5, -25) -> (-26.5, -16.6667)
  line L3 (-26.5, -16.6667) -> (-32, -16.6667)
  line L4 (-32, -16.6667) -> (-32, -25)
  line L5 (-1026.854, 0) -> (1026.854, 0) projected
  line L6 (-32, 25) -> (-26.5, 25)
  line L7 (-26.5, 25) -> (-26.5, 16.6667)
  line L8 (-26.5, 16.6667) -> (-32, 16.6667)
  line L9 (-32, 16.6667) -> (-32, 25)
  line L10 (32, -25) -> (26.5, -25)
  line L11 (26.5, -25) -> (26.5, -16.6667)
  line L12 (26.5, -16.6667) -> (32, -16.6667)
  line L13 (32, -16.6667) -> (32, -25)
  line L14 (26.5, 25) -> (26.5, 16.6667)
  line L15 (32, 25) -> (26.5, 25)
  line L16 (26.5, 16.6667) -> (32, 16.6667)
  line L17 (32, 16.6667) -> (32, 25)
  point P0 (0, 0)
  dimension "d47" = 5.5
  dimension "d48" = 8.3333
  constraints: 32 end point, 9 symmetric about line, 2 parallel, 1 horizontal, 1 perpendicular
  measures "d47" distance of L2.end L3.end
  measures "d48" distance of L1.end L2.end
extrude "Extrusion10" cut sketch "Sketch7" against normal through all
sketch "Sketch8" plane through (0, 5.5, 0) normal (0, 1, 0) x (1, 0, 0)
  line L0 (-32, -16.6667) -> (-23, -16.6667)
  line L1 (-1026.854, 0) -> (1026.854, 0) projected
  line L2 (0, 47.9488) -> (0, -48.9927) projected
  line L3 (-32, 16.6667) -> (-26.5, 16.6667)
  line L4 (-32, 16.6667) -> (-23, 16.6667)
  line L5 (-32, -16.6667) -> (-26.5, -16.6667)
  line L6 (-26.5, -16.6667) -> (-26.5, -6.6667)
  line L7 (-26.5, -6.6667) -> (-32, -6.6667)
  line L8 (-32, -6.6667) -> (-32, -16.6667)
  line L9 (-32, 16.6667) -> (-23, 16.6667)
  line L10 (-32, 16.6667) -> (-26.5, 16.6667)
  line L11 (-26.5, 16.6667) -> (-26.5, 6.6667)
  line L12 (-26.5, 6.6667) -> (-32, 6.6667)
  line L13 (-32, 6.6667) -> (-32, 16.6667)
  line L14 (32, -16.6667) -> (23, -16.6667)
  line L15 (32, 16.6667) -> (23, 16.6667)
  line L16 (32, 16.6667) -> (23, 16.6667)
  line L17 (32, 16.6667) -> (26.5, 16.6667)
  line L18 (-32, -6.6667) -> (-26.5, -6.6667)
  line L19 (-26.5, 6.6667) -> (-32, 6.6667)
  line L20 (32, -16.6667) -> (23, -16.6667)
  line L21 (32, 16.6667) -> (26.5, 16.6667)
  line L22 (32, 16.6667) -> (23, 16.6667)
  line L23 (32, -16.6667) -> (26.5, -16.6667)
  line L24 (26.5, -16.6667) -> (26.5, -6.6667)
  line L25 (26.5, -6.6667) -> (32, -6.6667)
  line L26 (32, -6.6667) -> (32, -16.6667)
  line L27 (26.5, 16.6667) -> (26.5, 6.6667)
  line L28 (32, 16.6667) -> (23, 16.6667)
  line L29 (32, 16.6667) -> (26.5, 16.6667)
  line L30 (32, 6.6667) -> (32, 16.6667)
  line L31 (26.5, 6.6667) -> (32, 6.6667)
  line L32 (32, -6.6667) -> (26.5, -6.6667)
  line L33 (26.5, 6.6667) -> (32, 6.6667)
  line L34 (-26.5, -6.6667) -> (-32, -6.6667)
  line L35 (-32, -6.6667) -> (-32, 6.6667)
  line L36 (-32, 6.6667) -> (-26.5, 6.6667)
  line L37 (-26.5, 6.6667) -> (-26.5, -6.6667)
  line L38 (32, -6.6667) -> (26.5, -6.6667)
  line L39 (26.5, -6.6667) -> (26.5, 6.6667)
  line L40 (26.5, 6.6667) -> (32, 6.6667)
  line L41 (32, 6.6667) -> (32, -6.6667)
  point P0 (-26.5, -16.6667)
  point P1 (0, 0)
  point P2 (26.5, -16.6667)
  point P3 (26.5, -16.6667)
  dimension "d53" = 5.5
  dimension "d54" = 10
  dimension "d76" = 0.08
  constraints: 80 end point, 29 symmetric about line, 7 parallel, 5 horizontal, 3 perpendicular, 1 collinear
  measures "d53" distance of L6.end L7.end
  measures "d54" distance of L5.end L6.end
extrude "Extrusion11" cut sketch "Sketch8" against normal through all contours L35 L1 L37 L7 | L35 L12 L37 L1 | L39 L31 L41 L1 | L1 L41 L25 L39
equation "\"d37\" = Wt"
equation "\"d51\" = Wt"
equation "\"d58\" = d59"
equation "\"d60\" = d62"
equation "\"d61\" = d63"
equation "\"d64\" = d68"
equation "\"d65\" = d69"
equation "\"d66\" = d70"
equation "\"d67\" = d71"
equation "\"d2\" = Wt"
equation "\"d9\" = Wt"
equation "\"d12\" = Wt"
equation "\"d47\" = Wt"
equation "\"d48\" = 0.166667 * d1"
equation "\"d49\" = Wt"
equation "\"d53\" = Wt"
equation "\"d54\" = 0.2 * d1"
equation "\"d55\" = Wt"
equation "\"d76\" = Kerf"
equation "\"Wt\" = 5.5"
equation "\"d59\" = 0.1"
equation "\"d62\" = 0.1"
equation "\"d63\" = 0.1"
equation "\"d68\" = 0.1"
equation "\"d69\" = 0.1"
equation "\"d70\" = 0.1"
equation "\"d71\" = 0.1"
equation "\"Kerf\" = 0.08"
body "Solid1"
